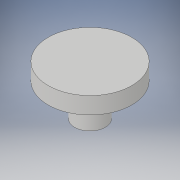
# Autodesk Inventor part: Grabber Base
Saved by Autodesk Inventor 2019.4 (Build 234330000, 330)
## iProperties
Created: 2020-12-03
Part Number: Grabber Base
Material: Generic
Document SubType Name: Modeling
Designer: caleb
Density: 1 g/cm^3
Appearance: Default
Author: caleb
Autodesk Inventor part; units mm, degrees
ref_plane "YZ Plane" through (0, 0, 0) normal (1, 0, 0) x (0, 1, 0)
ref_plane "XZ Plane" through (0, 0, 0) normal (0, 1, 0) x (-1, 0, 0)
ref_plane "XY Plane" through (0, 0, 0) normal (0, 0, 1) x (1, 0, 0)
sketch "Sketch1" plane through (0, 0, 0) normal (0, 1, 0) x (-1, 0, 0)
  circle A0 centre (0, 0) radius 26.035
  dimension "d0" = 52.07
  constraints: 1 centre point, 1 coincident
  measures "d0" diameter of A0
extrude "Extrusion1" add sketch "Sketch1" along normal blind 10.4648
sketch "Sketch2" plane through (0, 0, 0) normal (0, -1, 0) x (1, 0, 0)
  circle A0 centre (0, 0) radius 9.525
  dimension "d3" = 19.05
  constraints: 1 centre point, 1 coincident
  measures "d3" diameter of A0
extrude "Extrusion2" add sketch "Sketch2" along normal blind 20.32
sketch "Sketch3" plane through (0, -20.32, 0) normal (0, -1, 0) x (1, 0, 0)
  circle A0 centre (-4, 4) radius 1.5
  circle A1 centre (-4, -3.9878) radius 1.5
  circle A2 centre (3.9878, -3.9878) radius 1.5
  circle A3 centre (3.9878, 4) radius 1.5
  point P0 (0, 0)
  dimension "d6" = 4
  dimension "d7" = 4
  dimension "d8" = 3
  dimension "d9" = 3.9878
  dimension "d10" = 3.9878
  constraints: 4 centre point, 3 equal radius, 2 horizontal alignment, 2 vertical alignment
  measures "d6" horizontal distance of A0.centre point (0, 0)
  measures "d7" horizontal distance of point (0, 0) A0.centre
  measures "d8" diameter of A0
  measures "d9" vertical distance of A1.centre point (0, 0)
  measures "d10" horizontal distance of A2.centre point (0, 0)
hole "Hole1" at (-4, -20.32, -3.9878) at (-4, -20.32, 4) at (3.9878, -20.32, 4) at (3.9878, -20.32, -3.9878) direction (0, 1, 0) diameter 4.7625 depth 12.7 tip angle 118
body "Solid1"
